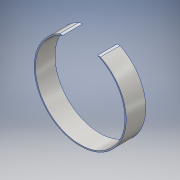
# Autodesk Inventor part: Cuerpo
Saved by Autodesk Inventor 2016 (Build 200138000, 138)
## iProperties
Created: 2019-03-15
Part Number: Cuerpo
Material: Aluminio 6061
Document SubType Name: Modeling
Designer: FIMCP
Mass: 69.3727 g
Surface Area: 276.138 cm^2
Volume: 25.6936 cm^3
Density: 2.7 g/cm^3
Appearance: Aluminio - Plano
Author: FIMCP
Autodesk Inventor part; units mm, degrees
ref_plane "YZ Plane" through (0, 0, 0) normal (1, 0, 0) x (0, 1, 0)
ref_plane "XZ Plane" through (0, 0, 0) normal (0, 1, 0) x (-1, 0, 0)
ref_plane "XY Plane" through (0, 0, 0) normal (0, 0, 1) x (1, 0, 0)
sketch "Boceto2" plane through (0, 0, 0) normal (0, 1, 0) x (-1, 0, 0)
  arc A0 (-18, 72.808) -> (20, 72.2842) centre (0, 0) ccw
  line L0 (-18, 72.808) -> (-18, 72.2842)
  line L1 (20, 72.2842) -> (13, 72.2842)
  line L2 (-18, 72.808) -> (-11, 72.808)
  line L3 (-11, 72.808) -> (-11, 72.2842)
  line L4 (-18, 72.2842) -> (-18, 72.808)
  line L5 (20, 72.2842) -> (13, 72.2842) projected
  line L6 (13, 72.2842) -> (20, 72.2842)
  line L7 (64.5832, 27.0002) -> (13, 27.0002)
  line L8 (13, 27.0002) -> (13, 72.2842)
  line L9 (-11, 72.2842) -> (-20, 72.2842)
  line L10 (-64.5832, 27.0002) -> (-11, 27.0002)
  line L11 (-11, 27.0002) -> (-11, 72.2842)
  arc A1 (69.8214, 4.9968) -> (69.8214, -4.9968) centre (70, 0) ccw
  arc A2 (-69.8214, -4.9968) -> (-69.8214, 4.9968) centre (-70, 0) ccw
  arc A3 (4.9968, -69.8214) -> (-4.9968, -69.8214) centre (0, -70) ccw
  arc A4 (4.9968, -69.8214) -> (69.8214, -4.9968) centre (0, 0) ccw
  arc A5 (69.8214, 4.9968) -> (64.5832, 27.0002) centre (0, 0) ccw
  arc A6 (-64.5832, 27.0002) -> (-69.8214, 4.9968) centre (0, 0) ccw
  arc A7 (-69.8214, -4.9968) -> (-4.9968, -69.8214) centre (0, 0) ccw
  dimension "d14" = 150
  dimension "d45" = 10
  dimension "d46" = 10
  dimension "d47" = 10
  constraints: 22 end point, 18 point on circle, 8 centre point, 4 horizontal, 3 parallel, 2 coincident, 2 point on line, 1 perpendicular
  measures "d14" diameter of A0
  measures "d45" diameter of A1
  measures "d46" diameter of A2
  measures "d47" diameter of A3
extrude "Extrusión2" add sketch "Boceto2" against normal blind 32 contours L9 L11 L10 A6 A2 A7 A3 A4 A1 A5 L7 L8 L1 A0
sketch "Boceto8" plane through (0, 0, 0) normal (0, 1, 0) x (-1, 0, 0)
  line L0 (59.5508, 67.2842) -> (-59.748, 67.2842)
  line L1 (-59.748, 67.2842) -> (-59.748, 82.2842)
  line L2 (-59.748, 82.2842) -> (59.5508, 82.2842)
  line L3 (59.5508, 82.2842) -> (59.5508, 67.2842)
  line L4 (13, 72.2842) -> (20, 72.2842) projected
  point P0 (0, 0)
  dimension "d67" = 15
  dimension "d71" = 5
  constraints: 8 end point, 2 parallel, 1 horizontal, 1 perpendicular
  measures "d67" distance of L0.end L1.end
  measures "d71" distance between parallel lines of L4 L0
extrude "Extrusión8" cut sketch "Boceto8" along normal mid plane 70
sketch "Boceto9" plane through (0, 0, 0) normal (0, 1, 0) x (-1, 0, 0)
  line L0 (-64.5832, 27.0002) -> (-11, 27.0002) projected
  line L1 (-23, 27.0002) -> (-64.5832, 27.0002)
  line L2 (-40.2309, 57.2842) -> (-23, 57.2842)
  line L3 (-23, 57.2842) -> (-23, 27.0002)
  line L4 (-11, 67.2842) -> (-11, 27.0002) projected
  line L5 (-33.1337, 67.2842) -> (-11, 67.2842) projected
  line L6 (25, 27.0002) -> (64.5832, 27.0002)
  line L7 (40.2309, 57.2842) -> (25, 57.2842)
  line L8 (25, 57.2842) -> (25, 27.0002)
  line L9 (13, 27.0002) -> (13, 67.2842) projected
  line L10 (13, 67.2842) -> (33.1337, 67.2842) projected
  arc A0 (-40.2309, 57.2842) -> (-64.5832, 27.0002) centre (0, 0) ccw
  arc A1 (64.5832, 27.0002) -> (40.2309, 57.2842) centre (0, 0) ccw
  dimension "d73" = 12
  dimension "d76" = 10
  dimension "d77" = 12
  dimension "d78" = 10
  constraints: 12 end point, 4 point on circle, 2 centre point, 2 horizontal, 2 parallel, 1 coincident, 1 point on line
  measures "d73" distance between parallel lines of L4 L3
  measures "d76" distance between parallel lines of L5 L2
  measures "d77" distance between parallel lines of L8 L9
  measures "d78" distance between parallel lines of L10 L7
extrude "Extrusión9" cut sketch "Boceto9" against normal blind 32
sketch "Boceto15" plane through (0, 0, 0) normal (0, 1, 0) x (-1, 0, 0)
  circle A0 centre (0, 0) radius 73
  dimension "d126" = 146
  constraints: 1 centre point, 1 coincident
  measures "d126" diameter of A0
extrude "Extrusión15" cut sketch "Boceto15" against normal blind 32
